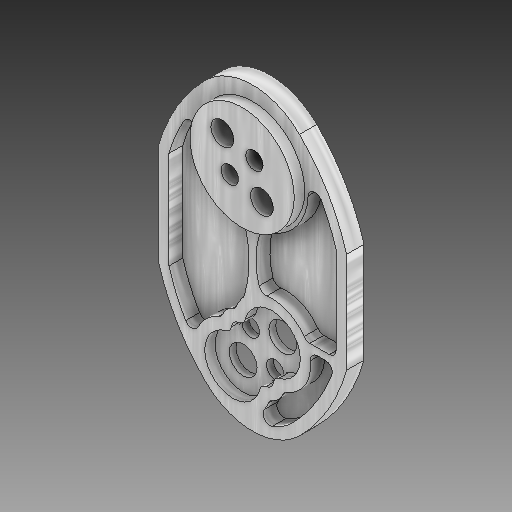
# Autodesk Inventor part: 脚クランクハッピーターン1
Saved by Autodesk Inventor 2020 (Build 240168000, 168)
## iProperties
Created: 2019-07-23
Part Number: 脚クランクハッピーターン1
Material: アルミニウム 7075
Document SubType Name: Modeling
Designer: 雪村
Density: 2.81 g/cm^3
Appearance: サテン - ブラシ仕上げ 重厚
Mass: 4.39464 g
Surface Area: 26.6095 cm^2
Volume: 1.56393 cm^3
Description: アルミ7000 4t
Author: 雪村
Autodesk Inventor part; units mm, degrees
ref_plane "YZ Plane" through (0, 0, 0) normal (1, 0, 0) x (0, 1, 0)
ref_plane "XZ Plane" through (0, 0, 0) normal (0, 1, 0) x (-1, 0, 0)
ref_plane "XY Plane" through (0, 0, 0) normal (0, 0, 1) x (1, 0, 0)
sketch "スケッチ1" plane through (0, 0, 0) normal (0, 0, 1) x (1, 0, 0)
  line L0 (-12.020815, -12.020815) -> (-12.020815, 12.020815)
  circle A0 centre (-14.86692, 14.86692) radius 2
  circle A1 centre (-9.17471, 9.17471) radius 2
  circle A2 centre (-13.788582, 10.253048) radius 1.25
  circle A3 centre (-10.253048, 13.788582) radius 1.25
  circle A4 centre (-14.86692, -14.86692) radius 4.025
  circle A5 centre (-9.17471, -9.17471) radius 4.025
  line L1 (-14.86692, -14.86692) -> (-9.17471, -9.17471)
  circle A6 centre (-9.17471, -9.17471) radius 2
  circle A7 centre (-14.86692, -14.86692) radius 2
  circle A8 centre (-13.788582, -10.253048) radius 1.25
  circle A9 centre (-10.253048, -13.788582) radius 1.25
  line L2 (-13.788582, -10.253048) -> (-10.253048, -13.788582)
  arc A10 (-9.574653, 16.453592) -> (-16.453592, 9.574653) centre (-14.86692, 14.86692) ccw
  circle A11 centre (-14.86692, -14.86692) radius 5.525
  circle A12 centre (-9.17471, 9.17471) radius 4.025
  circle A13 centre (-9.17471, 9.17471) radius 5.525
  circle A14 centre (-9.17471, -9.17471) radius 5.525
  circle A15 centre (-12.020815, 12.020815) radius 9.55
  circle A16 centre (-12.020815, -12.020815) radius 9.55
  arc A17 (-18.773685, 18.773685) -> (-18.773685, -18.773685) centre (0, 0) ccw
  arc A18 (-5.267946, -18.773685) -> (-5.267946, 18.773685) centre (-24.041631, 0) ccw
  point P0 (0, 0)
  point P1 (0, 0)
  point P2 (-9.346223, -14.648912)
  point P3 (-9.344531, -14.6971)
  point P4 (-9.392718, -14.695408)
  point P5 (-10.841993, -14.891145)
  point P6 (-14.891145, -10.841993)
  point P7 (-14.695408, -9.392718)
  point P8 (-14.6971, -9.344531)
  point P9 (-14.648912, -9.346223)
  point P10 (-12.615447, -9.821477)
  point P11 (-12.020815, -10.131383)
  point P12 (-10.980365, -12.771965)
  point P13 (-12.020815, -4.439173)
  point P14 (-12.020815, -2.470815)
  point P15 (-5.267946, -5.267946)
  point P16 (-13.081475, -13.081475)
  point P17 (-11.426184, -14.220153)
  point P18 (-11.269666, -13.061266)
  dimension "d0" = 8.05
  dimension "d1" = 8.05
  dimension "d2" = 4
  dimension "d3" = 4
  dimension "d4" = 2.5
  dimension "d5" = 2.5
  dimension "d6" = 5
  dimension "d7" = 1.5
  dimension "d8" = 8.05
  dimension "d9" = 1.5
  dimension "d10" = 1.5
  dimension "d11" = 26.55
  dimension "d12" = 26.55
  dimension "d13" = 24.04163
  constraints: 17 centre point, 10 point on circle, 6 end point, 6 tangent, 5 coincident, 3 midpoint, 1 perpendicular, 1 point on line, 1 vertical, 13 other
  measures "d2" diameter of A6
  measures "d3" diameter of A7
  measures "d4" diameter of A8
  measures "d5" diameter of A9
  measures "d6" distance of L2.start L2.end
  measures "d8" diameter of A12
  measures "d9" radial gap between concentric circles of A12 A13
  measures "d11" radius of A17
  measures "d12" radius of A18
  measures "d13" distance of L0.start L0.end
sketch "スケッチ1 outline for 押し出し1" plane through (0, 0, 0) normal (0, 0, 1) x (1, 0, 0)
  arc A0 (-18.773685, -18.773685) -> (-5.267946, -18.773685) centre (-12.020815, -12.020815) ccw
  arc A1 (-5.267946, -18.773685) -> (-5.267946, 18.773685) centre (-24.041631, 0) ccw
  arc A2 (-5.267946, 18.773685) -> (-18.773685, 18.773685) centre (-12.020815, 12.020815) ccw
  arc A3 (-18.773685, 18.773685) -> (-18.773685, -18.773685) centre (0, 0) ccw
  circle A4 centre (-10.253048, -13.788582) radius 1.25
  circle A5 centre (-13.788582, -10.253048) radius 1.25
  circle A6 centre (-9.17471, -9.17471) radius 2
  circle A7 centre (-13.788582, 10.253048) radius 1.25
  circle A8 centre (-14.86692, 14.86692) radius 2
  circle A9 centre (-9.17471, 9.17471) radius 2
  circle A10 centre (-10.253048, 13.788582) radius 1.25
  circle A11 centre (-14.86692, -14.86692) radius 2
extrude "押し出し1" add sketch "スケッチ1 outline for 押し出し1" along normal blind 4
sketch "スケッチ2" plane through (0, 0, 4) normal (0, 0, 1) x (1, 0, 0)
  circle A0 centre (-13.788582, -10.253048) radius 1.25
  circle A1 centre (-14.86692, -14.86692) radius 2
  circle A2 centre (-13.788582, 10.253048) radius 1.25
  circle A3 centre (-14.86692, 14.86692) radius 2
  circle A4 centre (-9.17471, -9.17471) radius 2
  circle A5 centre (-9.17471, 9.17471) radius 2
  circle A6 centre (-10.253048, 13.788582) radius 1.25
  arc A7 (-18.773685, 18.773685) -> (-18.773685, -18.773685) centre (0, 0) ccw
  arc A8 (-18.773685, -18.773685) -> (-5.267946, -18.773685) centre (-12.020815, -12.020815) ccw
  arc A9 (-5.267946, -18.773685) -> (-5.267946, 18.773685) centre (-24.041631, 0) ccw
  arc A10 (-5.267946, 18.773685) -> (-18.773685, 18.773685) centre (-12.020815, 12.020815) ccw
  circle A11 centre (-10.253048, -13.788582) radius 1.25
  circle A12 centre (-12.020815, 12.020815) radius 9.55
  circle A13 centre (-12.020815, -12.020815) radius 9.55
  circle A14 centre (-12.020815, 12.020815) radius 7.5
  point P0 (0, 0)
  dimension "d17" = 15
  constraints: 3 centre point, 3 coincident, 2 concentric
  measures "d17" diameter of A14
sketch "スケッチ2 outline for 押し出し2" plane through (0, 0, 4) normal (0, 0, 1) x (1, 0, 0)
  arc A0 (-5.267946, -18.773685) -> (-5.267946, 18.773685) centre (-24.041631, 0) ccw
  arc A1 (-18.773685, -18.773685) -> (-5.267946, -18.773685) centre (-12.020815, -12.020815) ccw
  arc A2 (-5.267946, 18.773685) -> (-18.773685, 18.773685) centre (-12.020815, 12.020815) ccw
  arc A3 (-18.773685, 18.773685) -> (-18.773685, -18.773685) centre (0, 0) ccw
  circle A4 centre (-14.86692, -14.86692) radius 2
  circle A5 centre (-9.17471, -9.17471) radius 2
  circle A6 centre (-12.020815, 12.020815) radius 7.5
extrude "押し出し2" cut sketch "スケッチ2 outline for 押し出し2" against normal blind 1.5
sketch "スケッチ3" plane through (-12.020815, 12.020815, 4) normal (0, 0, 1) x (1, 0, 0)
  circle A0 centre (-2.846105, 2.846105) radius 2
  circle A1 centre (2.846105, -2.846105) radius 2
  circle A2 centre (-2.846105, 2.846105) radius 1.65
  circle A3 centre (2.846105, -2.846105) radius 1.65
  point P0 (12.020815, -12.020815)
  dimension "d20" = 3.3
  dimension "d21" = 3.3
  constraints: 2 centre point, 2 coincident
  measures "d20" diameter of A2
  measures "d21" diameter of A3
sketch "スケッチ3 outline for 押し出し3" plane through (-12.020815, 12.020815, 4) normal (0, 0, 1) x (1, 0, 0)
  circle A0 centre (2.846105, -2.846105) radius 2
  circle A1 centre (2.846105, -2.846105) radius 1.65
  circle A2 centre (-2.846105, 2.846105) radius 2
  circle A3 centre (-2.846105, 2.846105) radius 1.65
extrude "押し出し3" add sketch "スケッチ3 outline for 押し出し3" against normal blind 4
sketch "スケッチ4" plane through (0, 0, 2.5) normal (0, 0, 1) x (1, 0, 0)
  circle A0 centre (-14.86692, -14.86692) radius 2
  circle A1 centre (-9.17471, -9.17471) radius 2
  arc A2 (-12.538582, -10.253048) -> (-12.538582, -10.253048) centre (-13.788582, -10.253048) ccw
  arc A3 (-9.003048, -13.788582) -> (-9.003048, -13.788582) centre (-10.253048, -13.788582) ccw
  circle A4 centre (-14.86692, -14.86692) radius 4.025
  circle A5 centre (-9.17471, -9.17471) radius 4.025
  circle A6 centre (-13.788582, -10.253048) radius 1.275
  circle A7 centre (-10.253048, -13.788582) radius 1.275
  point P0 (0, 0)
  point P1 (-13.19937, -9.122361)
  point P2 (-14.91927, -10.842261)
  point P3 (-10.842261, -14.91927)
  point P4 (-9.122361, -13.19937)
  dimension "d24" = 8.05
  dimension "d25" = 8.05
  dimension "d26" = 2.55
  dimension "d27" = 2.55
  constraints: 4 centre point, 4 coincident
  measures "d24" diameter of A4
  measures "d25" diameter of A5
  measures "d26" diameter of A6
  measures "d27" diameter of A7
sketch "スケッチ4 outline for 押し出し4" plane through (0, 0, 2.5) normal (0, 0, 1) x (1, 0, 0)
  arc A0 (-13.19937, -9.122361) -> (-14.91927, -10.842261) centre (-13.788582, -10.253048) ccw
  arc A1 (-9.122361, -13.19937) -> (-13.19937, -9.122361) centre (-9.17471, -9.17471) ccw
  arc A2 (-14.91927, -10.842261) -> (-10.842261, -14.91927) centre (-14.86692, -14.86692) ccw
  arc A3 (-10.842261, -14.91927) -> (-9.122361, -13.19937) centre (-10.253048, -13.788582) ccw
  circle A4 centre (-14.86692, -14.86692) radius 2
  circle A5 centre (-9.17471, -9.17471) radius 2
extrude "押し出し4" cut sketch "スケッチ4 outline for 押し出し4" against normal blind 1.5
fillet "フィレット1" radius 1 4 edges at (-13.1994, -9.1224, 1.75) (-14.9193, -10.8423, 1.75) (-9.1224, -13.1994, 1.75) (-10.8423, -14.9193, 1.75)
sketch "スケッチ5" plane through (0, 0, 2.5) normal (0, 0, 1) x (1, 0, 0)
  arc A0 (-18.773685, 18.773685) -> (-18.773685, -18.773685) centre (0, 0) ccw
  arc A1 (-5.267946, -18.773685) -> (-5.267946, 18.773685) centre (-24.041631, 0) ccw
  line L0 (-25.55, 13.645382) -> (-25.55, -17.582955)
  line L1 (1.508369, 20.859762) -> (1.508369, -16.359679)
  point P0 (0, 0)
  point P1 (1.508369, 7.218033)
  point P2 (1.508369, -7.218033)
  point P3 (-25.55, -7.218033)
  point P4 (-25.55, 7.218033)
  dimension "d31" = 1
  dimension "d32" = 1
  constraints: 4 end point, 2 vertical
  measures "d31" distance edge to line of A1 L1
  measures "d32" distance edge to line of A0 L0
sketch "スケッチ5 outline for 押し出し5" plane through (0, 0, 2.5) normal (0, 0, 1) x (1, 0, 0)
  line L0 (1.508369, 7.218033) -> (1.508369, -7.218033)
  arc A0 (1.508369, -7.218033) -> (1.508369, 7.218033) centre (-24.041631, 0) ccw
  line L1 (-25.55, -7.218033) -> (-25.55, 7.218033)
  arc A1 (-25.55, 7.218033) -> (-25.55, -7.218033) centre (0, 0) ccw
extrude "押し出し5" cut sketch "スケッチ5 outline for 押し出し5" against normal through all
sketch "スケッチ6" plane through (0, 0, 2.5) normal (0, 0, 1) x (1, 0, 0)
  arc A0 (-15.812515, -10.954571) -> (-10.954571, -15.812515) centre (-14.86692, -14.86692) ccw
  arc A1 (-15.812515, -10.954571) -> (-15.054538, -10.101455) centre (-16.047445, -9.982559) ccw
  arc A2 (-13.940175, -8.987092) -> (-15.054538, -10.101455) centre (-13.788582, -10.253048) ccw
  arc A3 (-13.940175, -8.987092) -> (-13.08706, -8.229116) centre (-14.059072, -7.994186) ccw
  arc A4 (-8.229116, -13.08706) -> (-13.08706, -8.229116) centre (-9.17471, -9.17471) ccw
  arc A5 (-8.229116, -13.08706) -> (-8.987092, -13.940175) centre (-7.994186, -14.059072) ccw
  arc A6 (-10.101455, -15.054538) -> (-8.987092, -13.940175) centre (-10.253048, -13.788582) ccw
  arc A7 (-10.101455, -15.054538) -> (-10.954571, -15.812515) centre (-9.982559, -16.047445) ccw
  arc A8 (-25.55, -7.218033) -> (-18.773685, -18.773685) centre (0, 0) ccw
  arc A9 (-18.773685, -18.773685) -> (-5.267946, -18.773685) centre (-12.020815, -12.020815) ccw
  arc A10 (-5.267946, -18.773685) -> (1.508369, -7.218033) centre (-24.041631, 0) ccw
  line L0 (1.508369, -7.218033) -> (1.508369, 7.218033)
  line L1 (-25.55, 7.218033) -> (-25.55, -7.218033)
  arc A11 (-18.773685, 18.773685) -> (-25.55, 7.218033) centre (0, 0) ccw
  arc A12 (-5.267946, 18.773685) -> (-18.773685, 18.773685) centre (-12.020815, 12.020815) ccw
  arc A13 (1.508369, 7.218033) -> (-5.267946, 18.773685) centre (-24.041631, 0) ccw
  circle A14 centre (-12.020815, 12.020815) radius 7.5
  circle A15 centre (-12.020815, 12.020815) radius 8
  line L2 (-24.05, 7.007139) -> (-24.05, -7.007139)
  arc A16 (-24.05, -7.007139) -> (-17.713025, -17.713025) centre (0, 0) ccw
  arc A17 (-17.713025, -17.713025) -> (-6.328606, -17.713025) centre (-12.020815, -12.020815) ccw
  arc A18 (-6.328606, -17.713025) -> (0.008369, -7.007139) centre (-24.041631, 0) ccw
  line L3 (0.008369, -7.007139) -> (0.008369, 7.007139)
  arc A19 (0.008369, 7.007139) -> (-6.328606, 17.713025) centre (-24.041631, 0) ccw
  arc A20 (-6.328606, 17.713025) -> (-17.713025, 17.713025) centre (-12.020815, 12.020815) ccw
  arc A21 (-17.713025, 17.713025) -> (-24.05, 7.007139) centre (0, 0) ccw
  arc A22 (-14.458532, -7.560133) -> (-16.481498, -9.583099) centre (-13.788582, -10.253048) ccw
  arc A23 (-16.481498, -9.583099) -> (-9.583099, -16.481498) centre (-14.86692, -14.86692) ccw
  arc A24 (-9.583099, -16.481498) -> (-7.560133, -14.458532) centre (-10.253048, -13.788582) ccw
  arc A25 (-7.560133, -14.458532) -> (-14.458532, -7.560133) centre (-9.17471, -9.17471) ccw
  circle A26 centre (-21.01492, 11.695112) radius 1
  circle A27 centre (-3.026711, 11.695112) radius 1
  point P0 (0, 0)
  point P1 (-20.383435, -14.56084)
  point P2 (-12.885177, -20.024276)
  point P3 (-2.152909, 12.181395)
  point P4 (-4.026056, 11.731301)
  point P5 (-20.015575, 11.731301)
  point P6 (-21.888721, 12.181395)
  dimension "d35" = 0.5
  dimension "d36" = 1.5
  dimension "d37" = 1.5
  dimension "d40" = 2
  dimension "d41" = 2
  constraints: 20 point on circle, 13 centre point, 4 end point, 4 tangent, 10 other
  measures "d35" radial gap between concentric circles of A14 A15
  measures "d36" radial gap between concentric circles of A11 A21
  measures "d37" radial gap between concentric circles of A4 A25
  measures "d40" diameter of A26
  measures "d41" diameter of A27
sketch "スケッチ6 outline for 押し出し6" plane through (0, 0, 2.5) normal (0, 0, 1) x (1, 0, 0)
  arc A0 (-16.481498, -9.583099) -> (-14.458532, -7.560133) centre (-13.788582, -10.253048) cw
  arc A1 (-20.383435, -14.56084) -> (-16.481498, -9.583099) centre (-14.86692, -14.86692) cw
  arc A2 (-24.05, -7.007139) -> (-20.383435, -14.56084) centre (0, 0) ccw
  line L0 (-24.05, 7.007139) -> (-24.05, -7.007139)
  arc A3 (-21.888721, 12.181395) -> (-24.05, 7.007139) centre (0, 0) ccw
  arc A4 (-20.015575, 11.731301) -> (-21.888721, 12.181395) centre (-21.01492, 11.695112) ccw
  arc A5 (-4.026056, 11.731301) -> (-20.015575, 11.731301) centre (-12.020815, 12.020815) cw
  arc A6 (-2.152909, 12.181395) -> (-4.026056, 11.731301) centre (-3.026711, 11.695112) ccw
  arc A7 (0.008369, 7.007139) -> (-2.152909, 12.181395) centre (-24.041631, 0) ccw
  line L1 (0.008369, -7.007139) -> (0.008369, 7.007139)
  arc A8 (-6.328606, -17.713025) -> (0.008369, -7.007139) centre (-24.041631, 0) ccw
  arc A9 (-12.885177, -20.024276) -> (-6.328606, -17.713025) centre (-12.020815, -12.020815) ccw
  arc A10 (-9.583099, -16.481498) -> (-12.885177, -20.024276) centre (-14.86692, -14.86692) cw
  arc A11 (-7.560133, -14.458532) -> (-9.583099, -16.481498) centre (-10.253048, -13.788582) cw
  arc A12 (-14.458532, -7.560133) -> (-7.560133, -14.458532) centre (-9.17471, -9.17471) cw
extrude "押し出し6" cut sketch "スケッチ6 outline for 押し出し6" against normal through all
fillet "フィレット2" radius 1 6 edges at (-12.8852, -20.0243, 1.25) (-9.5831, -16.4815, 1.25) (-7.5601, -14.4585, 1.25) (-16.4815, -9.5831, 1.25) (-14.4585, -7.5601, 1.25) (-20.3834, -14.5608, 1.25)
sketch "スケッチ8" plane through (-12.020815, 12.020815, 4) normal (0, 0, 1) x (1, 0, 0)
  arc A0 (1.676809, -30.060885) -> (2.289363, -28.925528) centre (-2.846105, -26.887735) ccw
  arc A1 (2.834464, -28.37119) -> (2.289363, -28.925528) centre (3.218859, -29.294359) ccw
  arc A2 (2.834464, -28.37119) -> (4.32956, -26.876094) centre (1.767767, -25.809398) ccw
  arc A3 (4.883897, -26.330993) -> (4.32956, -26.876094) centre (5.252728, -27.26049) ccw
  arc A4 (4.883897, -26.330993) -> (-2.289363, -19.157733) centre (2.846105, -21.195526) ccw
  arc A5 (-2.834464, -19.712071) -> (-2.289363, -19.157733) centre (-3.218859, -18.788902) ccw
  arc A6 (-2.834464, -19.712071) -> (-4.32956, -21.207167) centre (-1.767767, -22.273864) ccw
  arc A7 (-4.883897, -21.752268) -> (-4.32956, -21.207167) centre (-5.252728, -20.822771) ccw
  arc A8 (-4.883897, -21.752268) -> (-7.852858, -24.551489) centre (-2.846105, -26.887735) ccw
  arc A9 (-9.623086, -24.632082) -> (-7.852858, -24.551489) centre (-8.759058, -24.128639) ccw
  arc A10 (-12.029185, -19.027954) -> (-9.623086, -24.632082) centre (12.020815, -12.020815) ccw
  line L0 (-12.029185, -19.027954) -> (-12.029185, -5.013676)
  arc A11 (-9.867906, 0.16058) -> (-12.029185, -5.013676) centre (12.020815, -12.020815) ccw
  arc A12 (-7.99476, -0.289514) -> (-9.867906, 0.16058) centre (-8.994105, -0.325703) ccw
  arc A13 (-7.99476, -0.289514) -> (7.99476, -0.289514) centre (0, 0) ccw
  arc A14 (9.867906, 0.16058) -> (7.99476, -0.289514) centre (8.994105, -0.325703) ccw
  arc A15 (12.029185, -5.013676) -> (9.867906, 0.16058) centre (-12.020815, -12.020815) ccw
  line L1 (12.029185, -5.013676) -> (12.029185, -19.027954)
  arc A16 (5.69221, -29.73384) -> (12.029185, -19.027954) centre (-12.020815, -12.020815) ccw
  arc A17 (2.849398, -31.570471) -> (5.69221, -29.73384) centre (0, -24.041631) ccw
  arc A18 (1.676809, -30.060885) -> (2.849398, -31.570471) centre (2.495435, -30.635211) ccw
  line L2 (13.529185, -19.238848) -> (13.529185, -4.802782)
  arc A19 (13.529185, -4.802782) -> (6.75287, 6.75287) centre (-12.020815, -12.020815) ccw
  arc A20 (6.75287, 6.75287) -> (-6.75287, 6.75287) centre (0, 0) ccw
  arc A21 (-6.75287, 6.75287) -> (-13.529185, -4.802782) centre (12.020815, -12.020815) ccw
  line L3 (-13.529185, -4.802782) -> (-13.529185, -19.238848)
  arc A22 (-13.529185, -19.238848) -> (-6.75287, -30.7945) centre (12.020815, -12.020815) ccw
  arc A23 (-6.75287, -30.7945) -> (6.75287, -30.7945) centre (0, -24.041631) ccw
  arc A24 (6.75287, -30.7945) -> (13.529185, -19.238848) centre (-12.020815, -12.020815) ccw
  arc A25 (1.91936, -27.075353) -> (1.066244, -27.83333) centre (2.038257, -28.06826) ccw
  arc A26 (-3.791699, -22.975386) -> (1.066244, -27.83333) centre (-2.846105, -26.887735) ccw
  arc A27 (-3.791699, -22.975386) -> (-3.033723, -22.122271) centre (-4.02663, -22.003374) ccw
  arc A28 (-1.91936, -21.007908) -> (-3.033723, -22.122271) centre (-1.767767, -22.273864) ccw
  arc A29 (-1.91936, -21.007908) -> (-1.066244, -20.249931) centre (-2.038257, -20.015001) ccw
  arc A30 (3.791699, -25.107875) -> (-1.066244, -20.249931) centre (2.846105, -21.195526) ccw
  arc A31 (3.791699, -25.107875) -> (3.033723, -25.960991) centre (4.02663, -26.079887) ccw
  arc A32 (1.91936, -27.075353) -> (3.033723, -25.960991) centre (1.767767, -25.809398) ccw
  circle A33 centre (0, 0) radius 7.5
  line L4 (0, -7.5) -> (0, -17.436936)
  line L5 (12.722511, -19.027954) -> (7.477596, -19.027954)
  arc A34 (4.883897, -26.330993) -> (-2.289363, -19.157733) centre (2.846105, -21.195526) ccw
  arc A35 (-1.25, -17.487757) -> (-1.25, -7.90174) centre (-16.190285, -12.694749) ccw
  arc A36 (1.25, -7.90174) -> (1.25, -15.906095) centre (11.553283, -11.903918) ccw
  line L6 (12.722511, -18.527954) -> (7.477596, -18.527954)
  line L7 (12.722511, -19.527954) -> (7.477596, -19.527954)
  point P0 (12.020815, -12.020815)
  point P1 (8.113441, -19.527954)
  point P2 (11.877832, -19.527954)
  point P3 (12.029185, -18.527954)
  point P4 (7.684461, -18.527954)
  point P5 (1.25, -15.906095)
  point P6 (-1.25, -17.487757)
  dimension "d43" = 9.93694
  dimension "d44" = 0.80667
  dimension "d45" = 4.63149
  dimension "d46" = 1.25
  dimension "d47" = 1.25
  dimension "d48" = 1.25
  dimension "d49" = 1.25
  dimension "d50" = 0.5
  dimension "d51" = 0.5
  dimension "d52" = 0.5
  dimension "d53" = 0.5
  constraints: 8 end point, 8 point on circle, 4 parallel, 3 point on line, 2 centre point, 1 horizontal, 1 vertical, 1 vertical alignment, 1 other
  measures "d43" distance of L4.start L4.end
  measures "d44" distance from line of L2 L5.start
  measures "d45" horizontal distance of A30.centre L5.end
  measures "d46" distance from line of L4 A35.end
  measures "d47" distance from line of L4 A36.start
  measures "d48" horizontal distance of A35.start L4.end
  measures "d49" horizontal distance of A36.end L4.end
  measures "d50" distance edge to line of A36 L4
  measures "d51" distance edge to line of A35 L4
  measures "d52" distance between parallel lines of L5 L6
  measures "d53" distance between parallel lines of L5 L7
sketch "スケッチ8 outline for 押し出し7" plane through (-12.020815, 12.020815, 4) normal (0, 0, 1) x (1, 0, 0)
  line L0 (8.113441, -19.527954) -> (11.877832, -19.527954)
  arc A0 (7.684461, -18.527954) -> (8.113441, -19.527954) centre (2.846105, -21.195526) cw
  line L1 (12.029185, -18.527954) -> (7.684461, -18.527954)
  line L2 (12.029185, -19.027954) -> (12.029185, -18.527954)
  arc A1 (11.877832, -19.527954) -> (12.029185, -19.027954) centre (-12.020815, -12.020815) ccw
  arc A2 (1.25, -15.906095) -> (1.25, -7.90174) centre (11.553283, -11.903918) cw
  arc A3 (-1.25, -17.487757) -> (1.25, -15.906095) centre (2.846105, -21.195526) cw
  arc A4 (-1.25, -7.90174) -> (-1.25, -17.487757) centre (-16.190285, -12.694749) cw
  arc A5 (1.25, -7.90174) -> (-1.25, -7.90174) centre (0, 0) cw
extrude "押し出し7" add sketch "スケッチ8 outline for 押し出し7" against normal blind 4
sketch "スケッチ9" plane through (-12.020815, 12.020815, 4) normal (0, 0, 1) x (1, 0, 0)
  arc A0 (1.25, -15.906095) -> (-1.25, -17.487757) centre (2.846105, -21.195526) ccw
  arc A1 (1.25, -7.90174) -> (1.25, -15.906095) centre (11.553283, -11.903918) ccw
  arc A2 (-1.25, -7.90174) -> (1.25, -7.90174) centre (0, 0) ccw
  arc A3 (-1.25, -17.487757) -> (-1.25, -7.90174) centre (-16.190285, -12.694749) ccw
  arc A4 (11.877832, -19.527954) -> (12.029185, -19.027954) centre (-12.020815, -12.020815) ccw
  line L0 (12.029185, -19.027954) -> (12.029185, -18.527954)
  line L1 (12.029185, -18.527954) -> (7.684461, -18.527954)
  arc A5 (8.113441, -19.527954) -> (7.684461, -18.527954) centre (2.846105, -21.195526) ccw
  line L2 (8.113441, -19.527954) -> (11.877832, -19.527954)
  point P0 (12.020815, -12.020815)
sketch "スケッチ9 outline for 押し出し8" plane through (-12.020815, 12.020815, 4) normal (0, 0, 1) x (1, 0, 0)
  line L0 (8.113441, -19.527954) -> (11.877832, -19.527954)
  arc A0 (7.684461, -18.527954) -> (8.113441, -19.527954) centre (2.846105, -21.195526) cw
  line L1 (12.029185, -18.527954) -> (7.684461, -18.527954)
  line L2 (12.029185, -19.027954) -> (12.029185, -18.527954)
  arc A1 (11.877832, -19.527954) -> (12.029185, -19.027954) centre (-12.020815, -12.020815) ccw
  arc A2 (-1.25, -17.487757) -> (1.25, -15.906095) centre (2.846105, -21.195526) cw
  arc A3 (-1.25, -7.90174) -> (-1.25, -17.487757) centre (-16.190285, -12.694749) cw
  arc A4 (1.25, -7.90174) -> (-1.25, -7.90174) centre (0, 0) cw
  arc A5 (1.25, -15.906095) -> (1.25, -7.90174) centre (11.553283, -11.903918) cw
extrude "押し出し8" cut sketch "スケッチ9 outline for 押し出し8" against normal blind 1.5
fillet "フィレット3" radius 1 8 edges at (-13.2708, 4.1191, 1.25) (-10.7708, 4.1191, 1.25) (-13.2708, -5.4669, 1.25) (-10.7708, -3.8853, 1.25) (-3.9074, -7.5071, 1.25) (-4.3364, -6.5071, 1.25) (0.0084, -6.5071, 1.25) (-0.143, -7.5071, 1.25)
sketch "スケッチ10" plane through (0, 0, 0) normal (0, 0, -1) x (-1, 0, 0)
  arc A0 (3.678702, -8.609449) -> (7.136918, -14.310178) centre (9.17471, -9.17471) ccw
  arc A1 (7.691255, -14.855279) -> (7.136918, -14.310178) centre (6.768087, -15.239674) ccw
  arc A2 (7.691255, -14.855279) -> (9.186351, -16.350375) centre (10.253048, -13.788582) ccw
  arc A3 (9.731453, -16.904712) -> (9.186351, -16.350375) centre (8.801956, -17.273544) ccw
  arc A4 (9.731453, -16.904712) -> (10.344007, -18.04007) centre (14.86692, -14.86692) ccw
  arc A5 (9.171417, -19.549655) -> (10.344007, -18.04007) centre (9.52538, -18.614396) ccw
  arc A6 (6.328606, -17.713025) -> (9.171417, -19.549655) centre (12.020815, -12.020815) ccw
  arc A7 (0.611147, -8.860866) -> (6.328606, -17.713025) centre (24.041631, 0) ccw
  arc A8 (1.546496, -7.507139) -> (0.611147, -8.860866) centre (1.546496, -8.507139) ccw
  line L0 (1.546496, -7.507139) -> (2.68395, -7.507139)
  arc A9 (3.678702, -8.609449) -> (2.68395, -7.507139) centre (2.68395, -8.507139) ccw
  arc A10 (13.829553, 4.227968) -> (20.015575, 11.731301) centre (12.020815, 12.020815) ccw
  arc A11 (21.888721, 12.181395) -> (20.015575, 11.731301) centre (21.01492, 11.695112) ccw
  arc A12 (24.05, 7.007139) -> (21.888721, 12.181395) centre (0, 0) ccw
  line L1 (24.05, 7.007139) -> (24.05, -7.007139)
  arc A13 (21.643901, -12.611267) -> (24.05, -7.007139) centre (0, 0) ccw
  arc A14 (19.873673, -12.530673) -> (21.643901, -12.611267) centre (20.779873, -12.107823) ccw
  arc A15 (19.873673, -12.530673) -> (16.904712, -9.731453) centre (14.86692, -14.86692) ccw
  arc A16 (16.350375, -9.186351) -> (16.904712, -9.731453) centre (17.273544, -8.801956) ccw
  arc A17 (16.350375, -9.186351) -> (14.855279, -7.691255) centre (13.788582, -10.253048) ccw
  arc A18 (14.310178, -7.136918) -> (14.855279, -7.691255) centre (15.239674, -6.768087) ccw
  arc A19 (14.310178, -7.136918) -> (13.397923, -5.612394) centre (9.17471, -9.17471) ccw
  arc A20 (13.205973, -5.259912) -> (13.397923, -5.612394) centre (14.162305, -4.96763) ccw
  arc A21 (13.092053, 3.521236) -> (13.205973, -5.259912) centre (28.211101, -0.673933) ccw
  arc A22 (13.829553, 4.227968) -> (13.092053, 3.521236) centre (14.055646, 3.253862) ccw
  line L2 (3.777994, -6.507139) -> (0.991631, -6.507139)
  arc A23 (-0.008369, -5.507139) -> (0.991631, -6.507139) centre (0.991631, -5.507139) ccw
  line L3 (-0.008369, -5.507139) -> (-0.008369, 7.007139)
  arc A24 (2.152909, 12.181395) -> (-0.008369, 7.007139) centre (24.041631, 0) ccw
  arc A25 (4.026056, 11.731301) -> (2.152909, 12.181395) centre (3.026711, 11.695112) ccw
  arc A26 (4.026056, 11.731301) -> (10.243688, 4.220699) centre (12.020815, 12.020815) ccw
  arc A27 (10.971885, 3.556905) -> (10.243688, 4.220699) centre (10.021547, 3.245684) ccw
  arc A28 (11.072407, -2.999462) -> (10.971885, 3.556905) centre (0.467532, 0.116897) ccw
  arc A29 (9.96918, -3.707129) -> (11.072407, -2.999462) centre (10.112975, -2.717522) ccw
  arc A30 (9.96918, -3.707129) -> (4.605077, -6.069219) centre (9.17471, -9.17471) ccw
  arc A31 (3.777994, -6.507139) -> (4.605077, -6.069219) centre (3.777994, -5.507139) ccw
  circle A32 centre (10.253048, -13.788582) radius 1.25
  line L4 (-1.508369, 7.218033) -> (-1.508369, -7.218033)
  arc A33 (-1.508369, -7.218033) -> (5.267946, -18.773685) centre (24.041631, 0) ccw
  arc A34 (5.267946, -18.773685) -> (18.773685, -18.773685) centre (12.020815, -12.020815) ccw
  arc A35 (18.773685, -18.773685) -> (25.55, -7.218033) centre (0, 0) ccw
  line L5 (25.55, -7.218033) -> (25.55, 7.218033)
  arc A36 (25.55, 7.218033) -> (18.773685, 18.773685) centre (0, 0) ccw
  arc A37 (18.773685, 18.773685) -> (5.267946, 18.773685) centre (12.020815, 12.020815) ccw
  arc A38 (5.267946, 18.773685) -> (-1.508369, 7.218033) centre (24.041631, 0) ccw
  circle A39 centre (10.253048, 13.788582) radius 1.25
  circle A40 centre (9.17471, -9.17471) radius 2
  circle A41 centre (13.788582, 10.253048) radius 1.25
  circle A42 centre (14.86692, -14.86692) radius 2
  circle A43 centre (13.788582, -10.253048) radius 1.25
  circle A44 centre (14.86692, 14.86692) radius 1.65
  circle A45 centre (9.17471, 9.17471) radius 1.65
  point P0 (0, 0)
sketch "スケッチ10 outline for 押し出し9" plane through (0, 0, 0) normal (0, 0, -1) x (-1, 0, 0)
  arc A0 (7.691255, -14.855279) -> (7.136918, -14.310178) centre (6.768087, -15.239674) ccw
  arc A1 (9.186351, -16.350375) -> (7.691255, -14.855279) centre (10.253048, -13.788582) cw
  arc A2 (9.731453, -16.904712) -> (9.186351, -16.350375) centre (8.801956, -17.273544) ccw
  arc A3 (10.344007, -18.04007) -> (9.731453, -16.904712) centre (14.86692, -14.86692) cw
  arc A4 (9.171417, -19.549655) -> (10.344007, -18.04007) centre (9.52538, -18.614396) ccw
  arc A5 (6.328606, -17.713025) -> (9.171417, -19.549655) centre (12.020815, -12.020815) ccw
  arc A6 (0.611147, -8.860866) -> (6.328606, -17.713025) centre (24.041631, 0) ccw
  arc A7 (1.546496, -7.507139) -> (0.611147, -8.860866) centre (1.546496, -8.507139) ccw
  line L0 (2.68395, -7.507139) -> (1.546496, -7.507139)
  arc A8 (3.678702, -8.609449) -> (2.68395, -7.507139) centre (2.68395, -8.507139) ccw
  arc A9 (7.136918, -14.310178) -> (3.678702, -8.609449) centre (9.17471, -9.17471) cw
  arc A10 (13.829553, 4.227968) -> (13.092053, 3.521236) centre (14.055646, 3.253862) ccw
  arc A11 (20.015575, 11.731301) -> (13.829553, 4.227968) centre (12.020815, 12.020815) cw
  arc A12 (21.888721, 12.181395) -> (20.015575, 11.731301) centre (21.01492, 11.695112) ccw
  arc A13 (24.05, 7.007139) -> (21.888721, 12.181395) centre (0, 0) ccw
  line L1 (24.05, -7.007139) -> (24.05, 7.007139)
  arc A14 (21.643901, -12.611267) -> (24.05, -7.007139) centre (0, 0) ccw
  arc A15 (19.873673, -12.530673) -> (21.643901, -12.611267) centre (20.779873, -12.107823) ccw
  arc A16 (16.904712, -9.731453) -> (19.873673, -12.530673) centre (14.86692, -14.86692) cw
  arc A17 (16.350375, -9.186351) -> (16.904712, -9.731453) centre (17.273544, -8.801956) ccw
  arc A18 (14.855279, -7.691255) -> (16.350375, -9.186351) centre (13.788582, -10.253048) cw
  arc A19 (14.310178, -7.136918) -> (14.855279, -7.691255) centre (15.239674, -6.768087) ccw
  arc A20 (13.397923, -5.612394) -> (14.310178, -7.136918) centre (9.17471, -9.17471) cw
  arc A21 (13.205973, -5.259912) -> (13.397923, -5.612394) centre (14.162305, -4.96763) ccw
  arc A22 (13.092053, 3.521236) -> (13.205973, -5.259912) centre (28.211101, -0.673933) ccw
  arc A23 (9.96918, -3.707129) -> (11.072407, -2.999462) centre (10.112975, -2.717522) ccw
  arc A24 (4.605077, -6.069219) -> (9.96918, -3.707129) centre (9.17471, -9.17471) cw
  arc A25 (3.777994, -6.507139) -> (4.605077, -6.069219) centre (3.777994, -5.507139) ccw
  line L2 (0.991631, -6.507139) -> (3.777994, -6.507139)
  arc A26 (-0.008369, -5.507139) -> (0.991631, -6.507139) centre (0.991631, -5.507139) ccw
  line L3 (-0.008369, 7.007139) -> (-0.008369, -5.507139)
  arc A27 (2.152909, 12.181395) -> (-0.008369, 7.007139) centre (24.041631, 0) ccw
  arc A28 (4.026056, 11.731301) -> (2.152909, 12.181395) centre (3.026711, 11.695112) ccw
  arc A29 (10.243688, 4.220699) -> (4.026056, 11.731301) centre (12.020815, 12.020815) cw
  arc A30 (10.971885, 3.556905) -> (10.243688, 4.220699) centre (10.021547, 3.245684) ccw
  arc A31 (11.072407, -2.999462) -> (10.971885, 3.556905) centre (0.467532, 0.116897) ccw
extrude "押し出し9" add sketch "スケッチ10 outline for 押し出し9" against normal blind 0.5
sketch "スケッチ14" plane through (0, 0, 0) normal (0, 0, -1) x (-1, 0, 0)
  circle A0 centre (13.788582, 10.253048) radius 1.25
  circle A1 centre (10.253048, 13.788582) radius 1.25
  point P0 (0, 0)
sketch "スケッチ14 outline for 押し出し11" plane through (0, 0, 0) normal (0, 0, -1) x (-1, 0, 0)
  circle A0 centre (10.253048, 13.788582) radius 1.25
  circle A1 centre (13.788582, 10.253048) radius 1.25
extrude "押し出し11" add sketch "スケッチ14 outline for 押し出し11" against normal blind 1
sketch "スケッチ16" plane through (-12.020815, 12.020815, 4) normal (0, 0, 1) x (1, 0, 0)
  circle A0 centre (2.846105, -2.846105) radius 1.65
  circle A1 centre (-2.846105, 2.846105) radius 1.65
  circle A2 centre (0, 0) radius 7.5
  circle A3 centre (-1.767767, -1.767767) radius 1.25
  circle A4 centre (1.767767, 1.767767) radius 1.25
  arc A5 (3.791699, -25.107875) -> (-1.066244, -20.249931) centre (2.846105, -21.195526) ccw
  arc A6 (-1.91936, -21.007908) -> (-1.066244, -20.249931) centre (-2.038257, -20.015001) ccw
  arc A7 (-1.91936, -21.007908) -> (-3.033723, -22.122271) centre (-1.767767, -22.273864) ccw
  arc A8 (-3.791699, -22.975386) -> (-3.033723, -22.122271) centre (-4.02663, -22.003374) ccw
  arc A9 (-3.791699, -22.975386) -> (1.066244, -27.83333) centre (-2.846105, -26.887735) ccw
  arc A10 (1.91936, -27.075353) -> (1.066244, -27.83333) centre (2.038257, -28.06826) ccw
  arc A11 (1.91936, -27.075353) -> (3.033723, -25.960991) centre (1.767767, -25.809398) ccw
  arc A12 (3.791699, -25.107875) -> (3.033723, -25.960991) centre (4.02663, -26.079887) ccw
  arc A13 (-2.834464, -19.712071) -> (-4.32956, -21.207167) centre (-1.767767, -22.273864) ccw
  arc A14 (-2.834464, -19.712071) -> (-2.289363, -19.157733) centre (-3.218859, -18.788902) ccw
  arc A15 (-1.377108, -17.633209) -> (-2.289363, -19.157733) centre (2.846105, -21.195526) ccw
  arc A16 (-1.377108, -17.633209) -> (-1.185158, -17.280727) centre (-2.14149, -16.988446) ccw
  arc A17 (-1.185158, -17.280727) -> (-1.071237, -8.499579) centre (-16.190285, -12.694749) ccw
  arc A18 (-1.071237, -8.499579) -> (-1.808738, -7.792847) centre (-2.03483, -8.766953) ccw
  arc A19 (-7.99476, -0.289514) -> (-1.808738, -7.792847) centre (0, 0) ccw
  arc A20 (-7.99476, -0.289514) -> (-9.867906, 0.16058) centre (-8.994105, -0.325703) ccw
  arc A21 (-9.867906, 0.16058) -> (-12.029185, -5.013676) centre (12.020815, -12.020815) ccw
  line L0 (-12.029185, -19.027954) -> (-12.029185, -5.013676)
  arc A22 (-12.029185, -19.027954) -> (-9.623086, -24.632082) centre (12.020815, -12.020815) ccw
  arc A23 (-9.623086, -24.632082) -> (-7.852858, -24.551489) centre (-8.759058, -24.128639) ccw
  arc A24 (-4.883897, -21.752268) -> (-7.852858, -24.551489) centre (-2.846105, -26.887735) ccw
  arc A25 (-4.883897, -21.752268) -> (-4.32956, -21.207167) centre (-5.252728, -20.822771) ccw
  line L1 (11.029185, -18.527954) -> (8.242821, -18.527954)
  arc A26 (11.029185, -18.527954) -> (12.029185, -17.527954) centre (11.029185, -17.527954) ccw
  line L2 (12.029185, -5.013676) -> (12.029185, -17.527954)
  arc A27 (12.029185, -5.013676) -> (9.867906, 0.16058) centre (-12.020815, -12.020815) ccw
  arc A28 (9.867906, 0.16058) -> (7.99476, -0.289514) centre (8.994105, -0.325703) ccw
  arc A29 (1.777128, -7.800117) -> (7.99476, -0.289514) centre (0, 0) ccw
  arc A30 (1.777128, -7.800117) -> (1.048931, -8.463911) centre (1.999269, -8.775131) ccw
  arc A31 (1.048931, -8.463911) -> (0.948408, -15.020277) centre (11.553283, -11.903918) ccw
  arc A32 (0.948408, -15.020277) -> (2.051636, -15.727945) centre (1.90784, -14.738337) ccw
  arc A33 (7.415738, -18.090034) -> (2.051636, -15.727945) centre (2.846105, -21.195526) ccw
  arc A34 (7.415738, -18.090034) -> (8.242821, -18.527954) centre (8.242821, -17.527954) ccw
  arc A35 (1.676809, -30.060885) -> (2.849398, -31.570471) centre (2.495435, -30.635211) ccw
  arc A36 (2.849398, -31.570471) -> (5.69221, -29.73384) centre (0, -24.041631) ccw
  arc A37 (5.69221, -29.73384) -> (11.409668, -20.881682) centre (-12.020815, -12.020815) ccw
  arc A38 (11.409668, -20.881682) -> (10.474319, -19.527954) centre (10.474319, -20.527954) ccw
  line L3 (9.336865, -19.527954) -> (10.474319, -19.527954)
  arc A39 (9.336865, -19.527954) -> (8.342113, -20.630264) centre (9.336865, -20.527954) ccw
  arc A40 (4.883897, -26.330993) -> (8.342113, -20.630264) centre (2.846105, -21.195526) ccw
  arc A41 (4.883897, -26.330993) -> (4.32956, -26.876094) centre (5.252728, -27.26049) ccw
  arc A42 (2.834464, -28.37119) -> (4.32956, -26.876094) centre (1.767767, -25.809398) ccw
  arc A43 (2.834464, -28.37119) -> (2.289363, -28.925528) centre (3.218859, -29.294359) ccw
  arc A44 (1.676809, -30.060885) -> (2.289363, -28.925528) centre (-2.846105, -26.887735) ccw
  circle A45 centre (1.767767, -25.809398) radius 1.25
  line L4 (13.529185, -4.802782) -> (13.529185, -19.238848)
  arc A46 (6.75287, -30.7945) -> (13.529185, -19.238848) centre (-12.020815, -12.020815) ccw
  arc A47 (-6.75287, -30.7945) -> (6.75287, -30.7945) centre (0, -24.041631) ccw
  arc A48 (-13.529185, -19.238848) -> (-6.75287, -30.7945) centre (12.020815, -12.020815) ccw
  line L5 (-13.529185, -19.238848) -> (-13.529185, -4.802782)
  arc A49 (-6.75287, 6.75287) -> (-13.529185, -4.802782) centre (12.020815, -12.020815) ccw
  arc A50 (6.75287, 6.75287) -> (-6.75287, 6.75287) centre (0, 0) ccw
  arc A51 (13.529185, -4.802782) -> (6.75287, 6.75287) centre (-12.020815, -12.020815) ccw
  circle A52 centre (2.846105, -21.195526) radius 2
  circle A53 centre (-2.846105, -26.887735) radius 2
  circle A54 centre (-1.767767, -22.273864) radius 1.25
  circle A55 centre (-2.846105, 2.846105) radius 1.65
  circle A56 centre (2.846105, -2.846105) radius 1.65
  point P0 (12.020815, -12.020815)
equation "\"d12\" = d11"
equation "\"d47\" = d46"
equation "\"d48\" = d46"
equation "\"d49\" = d47"
equation "\"d51\" = d50"
